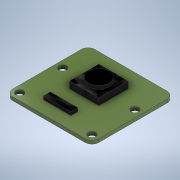
# Autodesk Inventor part: rpiCam
Saved by Autodesk Inventor 2020 (Build 240168000, 168)
## iProperties
Created: 2019-08-05
Part Number: rpiCam
Material: Generic
Document SubType Name: Modeling
Designer: n10208577
Density: 1 g/cm^3
Appearance: Default
Author: n10208577
Autodesk Inventor part; units mm, degrees
ref_plane "YZ Plane" through (0, 0, 0) normal (1, 0, 0) x (0, 1, 0)
ref_plane "XZ Plane" through (0, 0, 0) normal (0, 1, 0) x (-1, 0, 0)
ref_plane "XY Plane" through (0, 0, 0) normal (0, 0, 1) x (1, 0, 0)
sketch "Sketch1" plane through (0, 0, 0) normal (0, 1, 0) x (-1, 0, 0)
  line L0 (0, 0) -> (25, 0)
  line L1 (25, 0) -> (25, -23.862)
  line L2 (25, -23.862) -> (0, -23.862)
  line L3 (0, -23.862) -> (0, 0)
  line L4 (0, 0) -> (0, -2)
  line L5 (0, -2) -> (2, -2)
  line L6 (25, 0) -> (25, -2)
  line L7 (25, -2) -> (23, -2)
  circle A0 centre (2, -2) radius 1.1
  circle A1 centre (23, -2) radius 1.1
  line L8 (0, -2) -> (0, -14.5)
  line L9 (0, -14.5) -> (2, -14.5)
  line L10 (23, -2) -> (23, -14.5)
  circle A2 centre (23, -14.5) radius 1.1
  circle A3 centre (2, -14.5) radius 1.1
  dimension "d0" = 25
  dimension "d1" = 23.862
  dimension "d2" = 2
  dimension "d3" = 2
  dimension "d4" = 2
  dimension "d5" = 2
  dimension "d6" = 2.2
  dimension "d7" = 2.2
  dimension "d8" = 12.5
  dimension "d9" = 2
  dimension "d10" = 12.5
  dimension "d11" = 2.2
  dimension "d12" = 2.2
  constraints: 22 end point, 4 centre point, 4 coincident, 4 perpendicular, 3 point on line, 2 parallel, 1 horizontal, 1 vertical
  measures "d0" distance of L1.end L2.end
  measures "d1" distance of L0.end L1.end
  measures "d2" distance of L0.start L4.end
  measures "d3" distance of L4.end L5.end
  measures "d4" distance of L0.end L6.end
  measures "d5" distance of L6.end L7.end
  measures "d6" diameter of A0
  measures "d7" diameter of A1
  measures "d8" distance of L4.end L8.end
  measures "d9" distance of L8.end L9.end
  measures "d10" distance of L10.start L10.end
  measures "d11" diameter of A2
  measures "d12" diameter of A3
extrude "Extrusion1" add sketch "Sketch1" along normal blind 1
fillet "Fillet1" radius 2 4 edges at (0, 0.5, 0) (0, 0.5, -23.862) (-25, 0.5, -23.862) (-25, 0.5, 0)
sketch "Sketch2" plane through (0, 1, 0) normal (0, 1, 0) x (1, 0, 0)
  arc A0 (-25, 2) -> (-23, 0) centre (-23, 2) ccw projected
  line L0 (-23, 0) -> (-2, 0) projected
  arc A1 (-2, 0) -> (0, 2) centre (-2, 2) ccw projected
  line L1 (0, 2) -> (0, 21.862) projected
  arc A2 (0, 21.862) -> (-2, 23.862) centre (-2, 21.862) ccw projected
  line L2 (-2, 23.862) -> (-23, 23.862) projected
  arc A3 (-23, 23.862) -> (-25, 21.862) centre (-23, 21.862) ccw projected
  line L3 (-25, 21.862) -> (-25, 2) projected
  circle A4 centre (-23, 14.5) radius 1.1 projected
  circle A5 centre (-23, 2) radius 1.1 projected
  circle A6 centre (-2, 14.5) radius 1.1 projected
  circle A7 centre (-2, 2) radius 1.1 projected
  circle A8 centre (-23, 14.5) radius 1.1 projected
  circle A9 centre (-2, 14.5) radius 1.1 projected
  line L4 (-23, 14.5) -> (-2, 14.5)
  line L5 (-12.5, 14.5) -> (-16.75, 14.5)
  line L6 (-16.75, 14.5) -> (-16.75, 10.25)
  line L7 (-16.75, 10.25) -> (-8.25, 10.25)
  line L8 (-8.25, 10.25) -> (-8.25, 18.75)
  line L9 (-8.25, 18.75) -> (-16.75, 18.75)
  line L10 (-16.75, 18.75) -> (-16.75, 10.25)
  point P0 (0, 0)
  dimension "d16" = 4.25
  dimension "d17" = 4.25
  dimension "d18" = 8.5
  dimension "d19" = 8.5
  constraints: 14 end point, 2 horizontal, 2 parallel, 2 perpendicular, 1 midpoint, 1 point on line
  measures "d16" distance of L5.start L5.end
  measures "d17" distance of L5.end L6.end
  measures "d18" distance of L9.end L8.end
  measures "d19" distance of L8.end L7.end
extrude "Extrusion2" add sketch "Sketch2" along normal blind 2 contours L10 L9 L8 L4 | L4 L8 L7 L6
sketch "Sketch3" plane through (0, 3, 0) normal (0, 1, 0) x (1, 0, 0)
  line L0 (-16.75, 18.75) -> (-16.75, 10.25) projected
  line L1 (-16.75, 10.25) -> (-8.25, 10.25) projected
  line L2 (-8.25, 10.25) -> (-8.25, 18.75) projected
  line L3 (-8.25, 18.75) -> (-16.75, 18.75) projected
  circle A0 centre (-12.5, 14.5) radius 3
  point P0 (0, 0)
  dimension "d22" = 6
  constraints: 1 centre point
  measures "d22" diameter of A0
extrude "Extrusion3" add sketch "Sketch3" along normal blind 1 contours A0
sketch "Sketch4" plane through (0, 1, 0) normal (0, 1, 0) x (1, 0, 0)
  line L0 (-16.75, 18.75) -> (-8.25, 18.75) projected
  line L1 (-8.25, 18.75) -> (-8.25, 10.25) projected
  line L2 (-8.25, 10.25) -> (-16.75, 10.25) projected
  line L3 (-16.75, 10.25) -> (-16.75, 18.75) projected
  arc A0 (-25, 2) -> (-23, 0) centre (-23, 2) ccw projected
  line L4 (-23, 0) -> (-2, 0) projected
  arc A1 (-2, 0) -> (0, 2) centre (-2, 2) ccw projected
  line L5 (0, 2) -> (0, 21.862) projected
  arc A2 (0, 21.862) -> (-2, 23.862) centre (-2, 21.862) ccw projected
  line L6 (-2, 23.862) -> (-23, 23.862) projected
  arc A3 (-23, 23.862) -> (-25, 21.862) centre (-23, 21.862) ccw projected
  line L7 (-25, 21.862) -> (-25, 2) projected
  circle A4 centre (-23, 14.5) radius 1.1 projected
  circle A5 centre (-23, 2) radius 1.1 projected
  circle A6 centre (-2, 14.5) radius 1.1 projected
  circle A7 centre (-2, 2) radius 1.1 projected
  line L8 (0, 0) -> (-13.8, 0)
  line L9 (-23, 0) -> (-2, 0) projected
  line L10 (-13.8, 0) -> (-13.8, 4.7)
  line L11 (-13.8, 4.7) -> (-9.8, 4.7)
  line L12 (-9.8, 4.7) -> (-9.8, 5.7)
  line L13 (-9.8, 5.7) -> (-17.8, 5.7)
  line L14 (-17.8, 5.7) -> (-17.8, 3.7)
  line L15 (-17.8, 3.7) -> (-9.8, 3.7)
  line L16 (-9.8, 3.7) -> (-9.8, 5.7)
  dimension "d25" = 13.8
  dimension "d26" = 4.7
  dimension "d27" = 4
  dimension "d28" = 1
  dimension "d29" = 8
  dimension "d30" = 2
  constraints: 16 end point, 3 perpendicular, 2 horizontal, 2 parallel, 1 point on line
  measures "d25" distance of L8.start L8.end
  measures "d26" distance of L8.end L10.end
  measures "d27" distance of L10.end L11.end
  measures "d28" distance of L11.end L12.end
  measures "d29" distance of L15.end L14.end
  measures "d30" distance of L14.end L13.end
extrude "Extrusion4" add sketch "Sketch4" along normal blind 1 contours L15 L14 L13 L12 L11 L10 | L10 L11 L16 L15
body "Solid1"
